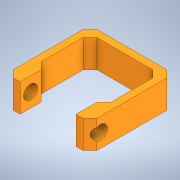
# Autodesk Inventor part: frame
Saved by Autodesk Inventor 2021 (Build 250183000, 183)
## iProperties
Created: 2022-05-14
Part Number: frame
Material: Generic
Document SubType Name: Modeling
Designer: ermoz
Density: 1 g/cm^3
Appearance: Default
Author: ermoz
Autodesk Inventor part; units mm, degrees
ref_plane "YZ Plane" through (0, 0, 0) normal (1, 0, 0) x (0, 1, 0)
ref_plane "XZ Plane" through (0, 0, 0) normal (0, 1, 0) x (-1, 0, 0)
ref_plane "XY Plane" through (0, 0, 0) normal (0, 0, 1) x (1, 0, 0)
sketch "Sketch1" plane through (0, 0, 0) normal (0, 1, 0) x (-1, 0, 0)
  line L0 (-60, -60) -> (60, -60)
  line L1 (60, -60) -> (60, 60)
  line L2 (60, 60) -> (-60, 60)
  line L3 (-60, 60) -> (-60, -60)
  line L4 (-60, -60) -> (60, 60) construction
  line L5 (60, -60) -> (-60, 60) construction
  line L6 (40, 60) -> (40, 30)
  line L7 (40, 30) -> (50, 30)
  line L8 (50, 30) -> (50, -50)
  line L9 (50, -50) -> (-50, -50)
  line L10 (-50, -50) -> (-50, 30)
  line L11 (-50, 30) -> (-40, 30)
  line L12 (-40, 30) -> (-40, 60)
  point P0 (0, 0)
  dimension "d0" = 120
  dimension "d1" = 120
  dimension "d2" = 20
  dimension "d3" = 20
  dimension "d4" = 10
  dimension "d5" = 10
  dimension "d6" = 10
  dimension "d7" = 30
  constraints: 26 end point, 7 perpendicular, 2 midpoint, 2 parallel, 2 point on line, 1 collinear, 1 horizontal, 1 vertical
  measures "d0" distance of L0.end L1.end
  measures "d1" distance of L1.end L2.end
  measures "d2" distance between parallel lines of L1 L6
  measures "d3" distance between parallel lines of L3 L12
  measures "d4" distance between parallel lines of L1 L8
  measures "d5" distance between parallel lines of L3 L10
  measures "d6" distance between parallel lines of L0 L9
  measures "d7" distance between parallel lines of L2 L7
extrude "Extrusion1" add sketch "Sketch1" along normal blind 40 contours L3 L2 L12 L11 L10 L9 L8 L7 L6 L1 L0
chamfer "Chamfer1" distance 10 angle 45 8 edges at (60, 20, 60) (60, 20, -60) (-50, 20, -50) (-60, 20, -60) (50, 20, -50) (-60, 20, 60) (50, 20, 30) (-50, 20, 30)
sketch "Sketch2" plane through (-60, 0, -50) normal (-1, 0, 0) x (0, 0, 1)
  circle A0 centre (95, 20) radius 10
  line L0 (110, 0) -> (110, 40) projected
  line L1 (0, 40) -> (100, 40) projected
  point P0 (50, 0)
  dimension "d13" = 15
  dimension "d14" = 20
  dimension "d15" = 20
  constraints: 1 centre point
  measures "d13" distance from line of L0 A0.centre
  measures "d14" diameter of A0
  measures "d15" distance from line of L1 A0.centre
extrude "Extrusion2" cut sketch "Sketch2" against normal through all
equation "\"d5\" = d4"
body "Solid1"
